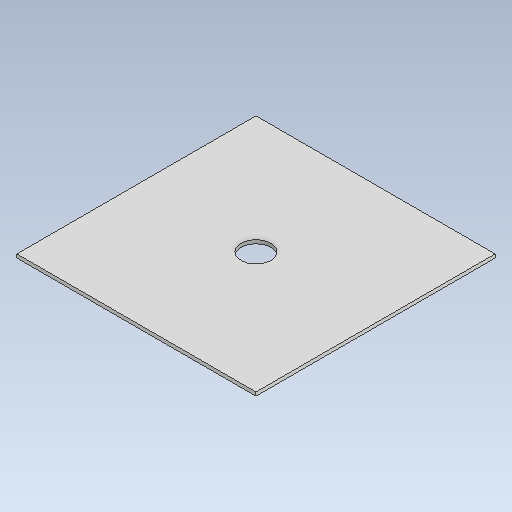
# Autodesk Inventor part: Днище
Saved by Autodesk Inventor 2020 (Build 240168000, 168)
## iProperties
Created: 2019-11-03
Part Number: Днище
Material: Типовые
Document SubType Name: Modeling
Designer: Михаил
Density: 1 g/cm^3
Appearance: По умолчанию
Author: Михаил
Autodesk Inventor part; units mm, degrees
ref_plane "YZ Plane" through (0, 0, 0) normal (1, 0, 0) x (0, 1, 0)
ref_plane "XZ Plane" through (0, 0, 0) normal (0, 1, 0) x (-1, 0, 0)
ref_plane "XY Plane" through (0, 0, 0) normal (0, 0, 1) x (1, 0, 0)
sketch "Эскиз1" plane through (0, 0, 0) normal (0, 1, 0) x (-1, 0, 0)
  line L0 (0, 0) -> (400, 0)
  line L1 (400, 0) -> (400, -400)
  line L2 (400, -400) -> (0, -400)
  line L3 (0, -400) -> (0, 0)
  dimension "d0" = 400
  dimension "d1" = 400
  constraints: 8 end point, 2 parallel, 1 horizontal, 1 perpendicular
  measures "d0" distance between parallel lines of L3 L1
  measures "d1" distance between parallel lines of L0 L2
extrude "Выдавливание1" add sketch "Эскиз1" along normal blind 6
sketch "Эскиз2" plane through (0, 6, 0) normal (0, 1, 0) x (1, 0, 0)
  circle A0 centre (-203, 203) radius 25
  line L0 (-400, 0) -> (0, 0) projected
  line L1 (0, 0) -> (0, 400) projected
  dimension "d4" = 50
  dimension "d5" = 203
  dimension "d6" = 203
  constraints: 1 centre point
  measures "d4" diameter of A0
  measures "d5" distance from line of L0 A0.centre
  measures "d6" distance from line of L1 A0.centre
extrude "Выдавливание2" cut sketch "Эскиз2" against normal blind 6
sketch "Эскиз3" plane through (0, 6, 0) normal (0, 1, 0) x (1, 0, 0)
  line L0 (-400, 0) -> (0, 0) projected
  line L1 (0, 0) -> (-3, 0)
  line L2 (-3, 0) -> (-3, 3)
  line L3 (-3, 3) -> (0, 3)
  line L4 (0, 3) -> (0, 0)
  line L5 (0, 0) -> (0, 400) projected
  line L6 (0, 400) -> (-3, 400)
  line L7 (-3, 400) -> (-3, 397)
  line L8 (-3, 397) -> (0, 397)
  line L9 (0, 397) -> (0, 400)
  line L10 (-400, 400) -> (-400, 0) projected
  line L11 (-400, 400) -> (-397, 400)
  line L12 (-397, 400) -> (-397, 397)
  line L13 (-397, 397) -> (-400, 397)
  line L14 (-400, 397) -> (-400, 400)
  line L15 (-400, 0) -> (-397, 0)
  line L16 (-397, 0) -> (-397, 3)
  line L17 (-397, 3) -> (-400, 3)
  line L18 (-400, 3) -> (-400, 0)
  point P0 (0, 397)
  point P1 (-400, 3)
  point P2 (-397, 0)
  dimension "d9" = 3
  dimension "d10" = 3
  dimension "d11" = 3
  dimension "d12" = 3
  dimension "d13" = 3
  dimension "d14" = 3
  dimension "d15" = 3
  constraints: 32 end point, 8 parallel, 4 horizontal, 4 perpendicular, 3 point on line
  measures "d9" distance between parallel lines of L12 L14
  measures "d10" distance between parallel lines of L11 L13
  measures "d11" distance between parallel lines of L9 L7
  measures "d12" distance between parallel lines of L6 L8
  measures "d13" distance between parallel lines of L0 L3
  measures "d14" distance between parallel lines of L0 L17
  measures "d15" distance between parallel lines of L10 L16
